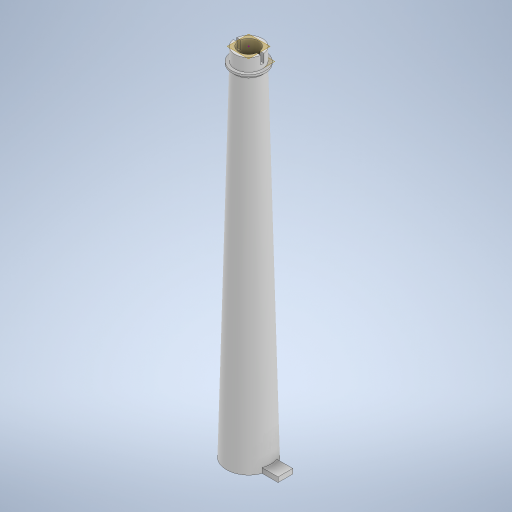
# Autodesk Inventor part: stozar
Saved by Autodesk Inventor 2023 (Build 270158000, 158)
## iProperties
Created: 2023-09-16
Part Number: stozar
Material: Generic
Document SubType Name: Modeling
Designer: alexa
Density: 1 g/cm^3
Appearance: Default
Author: alexa
Autodesk Inventor part; units mm, degrees
ref_plane "YZ Plane" through (0, 0, 0) normal (1, 0, 0) x (0, 1, 0)
ref_plane "XZ Plane" through (0, 0, 0) normal (0, 1, 0) x (-1, 0, 0)
ref_plane "XY Plane" through (0, 0, 0) normal (0, 0, 1) x (1, 0, 0)
sketch "Sketch11" plane through (0, 0, 0) normal (0, 1, 0) x (-1, 0, 0)
  circle A0 centre (0, 0) radius 14
  dimension "d24" = 28
  constraints: 1 centre point, 1 coincident
  measures "d24" diameter of A0
sketch "Sketch12" plane through (0, 0, 0) normal (0, 1, 0) x (-1, 0, 0)
  circle A0 centre (0, 0) radius 22.5
  line L0 (-105, -105) -> (105, -105)
  line L1 (105, -105) -> (105, 105)
  line L2 (105, 105) -> (-105, 105)
  line L3 (-105, 105) -> (-105, -105)
  line L4 (-105, -105) -> (105, 105) construction
  line L5 (105, -105) -> (-105, 105) construction
  dimension "d25" = 45
  dimension "d37" = 210
  dimension "d38" = 210
  constraints: 12 end point, 2 midpoint, 2 parallel, 1 centre point, 1 coincident, 1 horizontal, 1 perpendicular
  measures "d25" diameter of A0
  measures "d37" distance of L1.end L2.end
  measures "d38" distance of L0.end L1.end
extrude "Extrusion3" add sketch "Sketch11" along normal blind 350
loft "Loft4" add profiles "Sketch12" section 2 edges at (14, 350, 0) contours A0
sketch "Sketch13" plane through (0, 350, 0) normal (0, 1, 0) x (1, 0, 0)
  circle A0 centre (0, 0) radius 10
  dimension "d32" = 20
  constraints: 1 centre point, 1 coincident
  measures "d32" diameter of A0
sketch "Sketch14" plane through (0, 0, 0) normal (0, -1, 0) x (1, 0, 0)
  circle A0 centre (0, 0) radius 10
  dimension "d39" = 20
  constraints: 1 centre point, 1 coincident
  measures "d39" diameter of A0
loft "Loft5" cut profiles "Sketch14", "Sketch13"
ref_plane "Work Plane3" through (0, 363, 0) normal (0, 1, 0) x (1, 0, 0)
sketch "Sketch18" plane through (0, 363, 0) normal (0, 1, 0) x (1, 0, 0)
  point P0 (0, 0)
ref_plane "Work Plane4" through (0, 363, 0) normal (0, 1, 0) x (1, 0, 0)
ref_plane "Work Plane2" through (0, 350, 0) normal (0, 1, 0) x (1, 0, 0)
sketch "Sketch20" plane through (0, 350, 0) normal (0, 1, 0) x (1, 0, 0)
  circle A0 centre (0, 0) radius 17
  circle A1 centre (0, 0) radius 14 projected
  dimension "d57" = 34
  constraints: 1 centre point, 1 coincident
  measures "d57" diameter of A0
extrude "Extrusion8" add sketch "Sketch20" against normal blind 2
sketch "Sketch21" plane through (0, 348, 0) normal (0, -1, 0) x (1, 0, 0)
  point P0 (0, 0)
chamfer "Chamfer1" distance 2.951 angle 45 1 edges at (14.0486, 348, 0)
sketch "Sketch22" plane through (0, 350, 0) normal (0, 1, 0) x (1, 0, 0)
  circle A0 centre (0, 0) radius 14
  circle A1 centre (0, 0) radius 10
  dimension "d65" = 28
  constraints: 2 centre point, 2 coincident
  measures "d65" diameter of A0
extrude "Extrusion9" add sketch "Sketch22" along normal blind 13
sketch "Sketch23" plane through (0, 363, 0) normal (0, 1, 0) x (1, 0, 0)
  line L0 (-15, -1.6) -> (15, -1.6)
  line L1 (15, -1.6) -> (15, 1.6)
  line L2 (15, 1.6) -> (-15, 1.6)
  line L3 (-15, 1.6) -> (-15, -1.6)
  line L4 (-15, -1.6) -> (15, 1.6) construction
  line L5 (15, -1.6) -> (-15, 1.6) construction
  circle A0 centre (0, 0) radius 14 projected
  circle A1 centre (0, 0) radius 10 projected
  point P0 (-9.8712, -1.6)
  point P1 (-9.8712, 1.6)
  point P2 (-13.9083, 1.6)
  point P3 (-13.9083, -1.6)
  point P4 (9.8712, 1.6)
  point P5 (9.8712, -1.6)
  point P6 (13.9083, -1.6)
  point P7 (13.9083, 1.6)
  dimension "d68" = 3.2
  dimension "d69" = 30
  constraints: 12 end point, 2 midpoint, 2 parallel, 1 horizontal, 1 perpendicular
  measures "d68" distance between parallel lines of L2 L0
  measures "d69" distance between parallel lines of L1 L3
extrude "Extrusion10" cut sketch "Sketch23" against normal blind 8.5 contours A0 L2 A1 L0 | L0 A1 L2 A0
sketch "Sketch25" plane through (0, 0, 0) normal (0, -1, 0) x (1, 0, 0)
  line L0 (37.5, 7.5) -> (7.5, 7.5)
  line L1 (7.5, 7.5) -> (7.5, -7.5)
  line L2 (7.5, -7.5) -> (37.5, -7.5)
  line L3 (37.5, -7.5) -> (37.5, 7.5)
  line L4 (37.5, 7.5) -> (7.5, -7.5) construction
  line L5 (7.5, 7.5) -> (37.5, -7.5) construction
  circle A0 centre (0, 0) radius 10 projected
  circle A1 centre (0, 0) radius 22.5 projected
  point P0 (22.5, 0)
  point P1 (21.2132, 7.5)
  point P2 (21.2132, -7.5)
  dimension "d76" = 0
  dimension "d77" = 22.5
  dimension "d78" = 15
  dimension "d80" = 15
  constraints: 12 end point, 2 midpoint, 2 parallel, 1 horizontal, 1 perpendicular, 1 other
  measures "d76" vertical distance of point (22.5, 0) point (0, 0)
  measures "d77" distance of point (0, 0) point (22.5, 0)
  measures "d78" distance of L2.end L0.start
  measures "d80" distance from line of L3 point (22.5, 0)
extrude "Extrusion11" add sketch "Sketch25" against normal blind 5 contours L3 L2 A1 L0
sketch "Sketch26" plane through (0, 0, 0) normal (0, -1, 0) x (1, 0, 0)
  line L0 (-12.35, 10.15) -> (-17.65, 10.15)
  line L1 (-17.65, 10.15) -> (-17.65, -10.15)
  line L2 (-17.65, -10.15) -> (-12.35, -10.15)
  line L3 (-12.35, -10.15) -> (-12.35, 10.15)
  line L4 (-12.35, 10.15) -> (-17.65, -10.15) construction
  line L5 (-17.65, 10.15) -> (-12.35, -10.15) construction
  point P0 (0, 0)
  point P1 (-15, 0)
  dimension "d83" = 15
  dimension "d84" = 20.3
  dimension "d85" = 5.3
  dimension "d10" = 70
  dimension "d72" = 5
  dimension "d73" = 15
  dimension "d74" = 17
  dimension "d75" = 2.5
  constraints: 12 end point, 2 midpoint, 2 parallel, 1 horizontal, 1 perpendicular
  measures "d83" distance of point (0, 0) point (-15, 0)
  measures "d84" distance of L0.end L1.end
  measures "d85" distance of L1.end L2.end
extrude "Extrusion12" cut sketch "Sketch26" against normal blind 2.3
body "Solid3"
